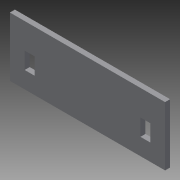
# Autodesk Inventor part: CNC-X-axis- front plate drawer exits
Saved by Autodesk Inventor 2015 (Build 190159000, 159)
## iProperties
Created: 2015-03-24
Part Number: CNC-X-axis- front plate drawer exits
Material: Generic
Document SubType Name: Modeling
Designer: Bangladesh
Density: 1 g/cm^3
Appearance: Default
Author: Bangladesh
Autodesk Inventor part; units mm, degrees
ref_plane "YZ Plane" through (0, 0, 0) normal (1, 0, 0) x (0, 1, 0)
ref_plane "XZ Plane" through (0, 0, 0) normal (0, 1, 0) x (-1, 0, 0)
ref_plane "XY Plane" through (0, 0, 0) normal (0, 0, 1) x (1, 0, 0)
sketch "Sketch1" plane through (0, 0, 0) normal (0, 0, 1) x (1, 0, 0)
  line L0 (-200, 76.2) -> (200, 76.2)
  line L1 (200, 76.2) -> (200, -76.2)
  line L2 (200, -76.2) -> (-200, -76.2)
  line L3 (-200, -76.2) -> (-200, 76.2)
  line L4 (-200, 76.2) -> (200, -76.2) construction
  line L5 (200, 76.2) -> (-200, -76.2) construction
  point P0 (0, 0)
  dimension "d0" = 400
  dimension "d1" = 152.4
  constraints: 12 end point, 2 midpoint, 2 parallel, 1 horizontal, 1 perpendicular
  measures "d0" distance of L1.end L2.end
  measures "d1" distance of L0.end L1.end
extrude "Extrusion1" add sketch "Sketch1" along normal mid plane 13
sketch "Sketch2" plane through (0, 0, 6.5) normal (0, 0, 1) x (1, 0, 0)
  line L0 (-161.9, 10.16) -> (-136.5, 10.16)
  line L1 (-136.5, 10.16) -> (-136.5, -33.02)
  line L2 (-136.5, -33.02) -> (-161.9, -33.02)
  line L3 (-161.9, -33.02) -> (-161.9, 10.16)
  line L4 (-200, -76.2) -> (200, -76.2) projected
  line L5 (161.9, -33.02) -> (136.5, -33.02)
  line L6 (136.5, -33.02) -> (136.5, 10.16)
  line L7 (136.5, 10.16) -> (161.9, 10.16)
  line L8 (161.9, 10.16) -> (161.9, -33.02)
  point P0 (0, 0)
  constraints: 16 end point, 4 parallel, 2 horizontal, 2 perpendicular
extrude "Extrusion2" cut sketch "Sketch2" against normal blind 13
body "Solid1"
